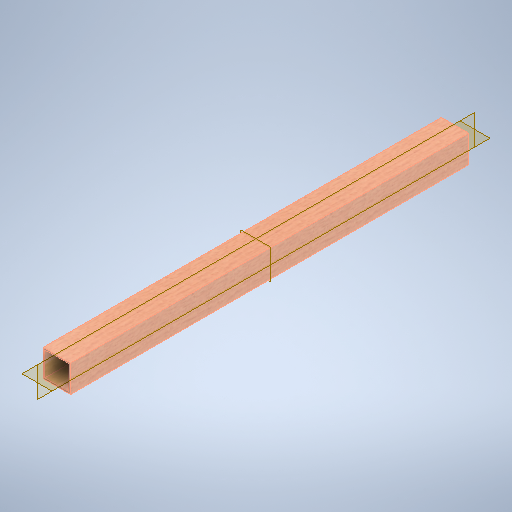
# Autodesk Inventor part: perna
Saved by Autodesk Inventor 2025.2 (Build 292293000, 293)
## iProperties
Created: 2025-04-02
Part Number: perna
Material: Wood (Walnut)
Document SubType Name: Modeling
Designer: kenne
Density: 0.55 g/cm^3
Appearance: White Oak - Natural Medium Gloss
Author: kenne
Autodesk Inventor part; units mm, degrees
sketch "Sketch1" plane through (0, 0, 0) normal (0, 0, 1) x (1, 0, 0)
  line L0 (-25, 25) -> (25, 25)
  line L1 (25, 25) -> (25, -25)
  line L2 (25, -25) -> (-25, -25)
  line L3 (-25, -25) -> (-25, 25)
  line L4 (-25, 25) -> (25, -25) construction
  line L5 (25, 25) -> (-25, -25) construction
  line L6 (-22, 22) -> (22, 22)
  line L7 (22, 22) -> (22, -22)
  line L8 (22, -22) -> (-22, -22)
  line L9 (-22, -22) -> (-22, 22)
  line L10 (-22, 22) -> (22, -22) construction
  line L11 (22, 22) -> (-22, -22) construction
  point P0 (0, 0)
  point P1 (0, 0)
  dimension "d0" = 50
  dimension "d1" = 3
  constraints: 24 end point, 4 midpoint, 4 parallel, 4 perpendicular, 2 horizontal, 1 coincident
  measures "d0" distance of L0.start L0.end
  measures "d1" distance between parallel lines of L0 L6
extrude "Extrusion1" add sketch "Sketch1" along normal mid plane 730
body "Solid1"
